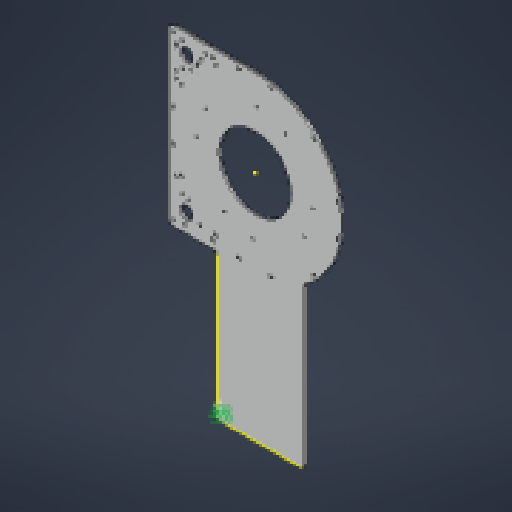
# Autodesk Inventor part: PLATE,SHOOTER,MOUNT
Saved by Autodesk Inventor 2026 (Build 300175000, 175)
## iProperties
Created: 2026-02-09
Part Number: PLATE,SHOOTER,MOUNT
Material: Aluminum 6061
Document SubType Name: Sheet Metal
Designer: littl
Density: 2.7 g/cm^3
Sheet Metal Rule: Default
Appearance: Aluminum - Flat
Mass: 776.002 g
Surface Area: 1574.73 cm^2
Volume: 287.408 cm^3
Author: littl
Autodesk Inventor part; units mm, degrees
ref_plane "YZ Plane" through (0, 0, 0) normal (1, 0, 0) x (0, 1, 0)
ref_plane "XZ Plane" through (0, 0, 0) normal (0, 1, 0) x (-1, 0, 0)
ref_plane "XY Plane" through (0, 0, 0) normal (0, 0, 1) x (1, 0, 0)
sketch "Sketch1" plane through (0, 0, 0) normal (0, 0, 1) x (1, 0, 0)
  line L0 (-190.5, -190.5) -> (190.5, -190.5)
  line L1 (190.5, -190.5) -> (190.5, 190.5)
  line L2 (190.5, 190.5) -> (-190.5, 190.5)
  line L3 (-190.5, 190.5) -> (-190.5, -190.5)
  line L4 (-190.5, -190.5) -> (190.5, 190.5) construction
  line L5 (190.5, -190.5) -> (-190.5, 190.5) construction
  circle A0 centre (0, 0) radius 79.375
  line L6 (130.599, -90.0738) -> (-0.5713, 156.6217) construction
  line L7 (-0.5713, 156.6217) -> (-129.5258, 88.0554) construction
  line L8 (-129.5258, 88.0554) -> (1.6445, -158.6401) construction
  line L9 (1.6445, -158.6401) -> (130.599, -90.0738) construction
  line L10 (130.599, -90.0738) -> (-129.5258, 88.0554) construction
  line L11 (-0.5713, 156.6217) -> (1.6445, -158.6401) construction
  line L12 (1.6445, -158.6401) -> (-64.4772, -34.2832) construction
  line L13 (-64.4772, -34.2832) -> (-12.5828, -6.6904) construction
  line L14 (-65.0486, 122.3386) -> (66.1218, -124.357) construction
  line L15 (-91.2837, -21.0636) -> (-75.8652, -12.8655) construction
  line L16 (-91.2837, -21.0636) -> (-85.3214, -32.2771) construction
  line L17 (-85.3214, -32.2771) -> (-79.3591, -43.4905) construction
  line L18 (68.5077, 63.899) -> (53.0893, 55.7008) construction
  line L19 (68.5077, 63.899) -> (74.47, 52.6855) construction
  line L20 (74.47, 52.6855) -> (80.4323, 41.4721) construction
  arc A1 (0, -190.5) -> (190.5, 0) centre (0, 0) ccw
  arc A2 (190.5, 0) -> (0, 190.5) centre (0, 0) ccw
  point P0 (0.5366, -1.0092)
  point P1 (152.4, 190.5)
  point P2 (-17.6976, -190.5)
  dimension "d0" = 381
  dimension "d1" = 158.75
  dimension "d2" = 279.4
  dimension "d3" = 146.05
  dimension "d4" = 28
  dimension "d5" = 140.843
  dimension "d6" = 114.3
  dimension "d7" = 17.4625
  dimension "d8" = 12.7
  dimension "d9" = 114.3
  dimension "d11" = 17.4625
  dimension "d12" = 12.7
  constraints: 42 end point, 9 midpoint, 7 coincident, 7 point on line, 6 parallel, 5 perpendicular, 4 point on circle, 3 centre point, 3 equal length, 2 collinear, 1 horizontal
  measures "d0" distance of L2.end L1.end
  measures "d1" diameter of A0
  measures "d2" distance of L6.start L6.end
  measures "d3" distance of L6.end L7.end
  measures "d4" angle of L3 L8
  measures "d5" distance of L8.end L12.end
  measures "d6" distance between parallel lines of L7 L15
  measures "d7" distance of L15.start L15.end
  measures "d8" distance of L15.start L16.end
  measures "d9" distance between parallel lines of L7 L18
  measures "d11" distance of L18.start L18.end
  measures "d12" distance of L19.end L20.end
extrude "Plate1" add sketch "Sketch1" along normal blind 4.7752 contours L3 L2 A2 A1 L0
fillet "Corner Round1" radius 12.7 2 edges at (-190.5, 190.5, 2.3876) (-190.5, -190.5, 2.3876)
sketch "Sketch7" plane through (0, 0, 4.7752) normal (0, 0, 1) x (1, 0, 0)
  line L0 (0, 0) -> (-126.9226, 4.4322) construction
  line L1 (0, 266.7) -> (0, -266.7) projected
  circle A0 centre (-79.3591, -43.4905) radius 2.4892 projected
  circle A1 centre (80.4323, 41.4721) radius 2.4892 projected
  line L2 (59.6229, -112.1343) -> (0, 0) construction
  circle A2 centre (-91.2837, -21.0636) radius 2.4892 projected
  circle A3 centre (68.5077, 63.899) radius 2.4892 projected
  line L3 (-91.2837, -21.0636) -> (-79.3591, -43.4905) construction
  line L4 (68.5077, 63.899) -> (80.4323, 41.4721) construction
  point P0 (-112.1343, -59.6229)
  point P1 (-67.2997, -107.7021)
  point P2 (-4.4322, -126.9226)
  point P3 (107.7021, -67.2997)
  point P4 (126.9226, -4.4322)
  point P5 (112.1343, 59.6229)
  point P6 (67.2997, 107.7021)
  point P7 (4.4322, 126.9226)
  point P8 (-59.6229, 112.1343)
  point P9 (-107.7021, 67.2997)
  dimension "d94" = 127
  dimension "d98" = 360
  constraints: 8 end point, 1 parallel, 13 other
  measures "d94" distance of L0.start L0.end
hole "Hole6" at (-126.9226, 4.4322, 4.7752) at (-67.2997, -107.7021, 4.7752) at (-4.4322, -126.9226, 4.7752) at (107.7021, -67.2997, 4.7752) at (126.9226, -4.4322, 4.7752) at (4.4322, 126.9226, 4.7752) at (67.2997, 107.7021, 4.7752) at (-107.7021, 67.2997, 4.7752) direction (0, 0, -1) diameter 4.9784 end through all thread size "1/4-20 UNC" class "2B" standard "ANSI Unified Screw Threads"
sketch "Sketch8" plane through (0, 0, 4.7752) normal (0, 0, 1) x (1, 0, 0)
  circle A0 centre (0, 0) radius 190.5 construction
  arc A1 (-177.8, 190.5) -> (-190.5, 177.8) centre (-177.8, 177.8) ccw projected
  line L0 (-177.8, 177.8) -> (0, 0) construction
  arc A2 (-190.5, -177.8) -> (-177.8, -190.5) centre (-177.8, -177.8) ccw projected
  line L1 (0, 0) -> (-177.8, -177.8) construction
  line L2 (-149.9703, -149.9703) -> (-172.4209, -172.4209) construction
  line L3 (-149.0723, 149.0723) -> (-171.5229, 171.5229) construction
  line L4 (-149.0723, 149.0723) -> (-123.9351, 145.4275) construction
  line L5 (-149.0723, 149.0723) -> (-128.558, 149.0723) construction
  line L6 (-149.9703, -149.9703) -> (-145.5596, -124.9562) construction
  line L7 (-149.9703, -149.9703) -> (-130.8542, -149.9703)
  line L8 (-177.8, 190.5) -> (0, 190.5) projected
  line L9 (-190.5, -177.8) -> (-190.5, 177.8) projected
  line L10 (0, -190.5) -> (-177.8, -190.5) projected
  point P0 (-119.3021, -158.1878)
  point P1 (-158.1878, -119.3021)
  point P2 (-157.2898, 118.4041)
  point P3 (-118.4041, 157.2898)
  point P4 (-174.2094, 152.717)
  point P5 (-154.3809, -174.9844)
  point P6 (-178.698, -178.698)
  dimension "d107" = 381
  dimension "d108" = 212.09
  dimension "d109" = 210.82
  dimension "d110" = 31.75
  dimension "d113" = 360
  dimension "d115" = 31.75
  dimension "d118" = 360
  dimension "d134" = 25.4
  dimension "d137" = 360
  dimension "d139" = 8.25
  dimension "d149" = 360
  dimension "d151" = 25.4
  dimension "d153" = 80
  dimension "d221" = 12.7
  dimension "d222" = 12.7
  dimension "d225" = 40.6272
  constraints: 16 end point, 3 point on line, 2 coincident, 2 collinear, 2 horizontal, 1 centre point, 1 perpendicular, 14 other
  measures "d107" diameter of A0
  measures "d108" distance of point (0, 0) L2.start
  measures "d109" distance of point (0, 0) L3.start
  measures "d110" distance of L2.start L2.end
  measures "d115" distance of L3.start L3.end
  measures "d134" distance of L3.start L4.end
  measures "d139" angle of L4 L5
  measures "d151" distance of L2.start L6.end
  measures "d153" angle of L7 L6
  measures "d221" distance from line of L8 point (-177.8, 177.8)
  measures "d222" distance from line of L9 point (-177.8, 177.8)
  measures "d225" distance of L2.start point (-178.698, -178.698)
hole "Hole7" at (-118.4041, 157.2898, 4.7752) at (-157.2898, 118.4041, 4.7752) at (-177.8, 177.8, 4.7752) at (-158.1878, -119.3021, 4.7752) at (-119.3021, -158.1878, 4.7752) at (-154.3809, -174.9844, 4.7752) at (-174.2094, 152.717, 4.7752) at (-178.698, -178.698, 4.7752) direction (0, 0, -1) diameter 6.5278 depth 4.7752 tip angle 118 clearance for "Flat Head Machine Screw (82)" size "1/4" standard "Ansi Unified Screw Threads"
hole "Hole8" at (-149.0723, 149.0723, 4.7752) at (-149.9703, -149.9703, 4.7752) direction (0, 0, -1) diameter 28.575 depth 4.7752 tip angle 118
hole "Hole9" at (-123.9351, 145.4275, 4.7752) at (-174.2094, 152.717, 4.7752) at (-154.3809, -174.9844, 4.7752) at (-145.5596, -124.9562, 4.7752) direction (0, 0, -1) diameter 4.9784 end through all clearance for "Flat Head Machine Screw (82)" size "#10" standard "Ansi Unified Screw Threads"
sketch "Sketch11" plane through (0, 0, 4.7752) normal (0, 0, 1) x (1, 0, 0)
  line L0 (179.674, -32.5022) -> (178.4352, -38.7302) construction
  line L1 (178.117, -32.1925) -> (176.8782, -38.4205)
  line L2 (179.9922, -39.0399) -> (181.231, -32.8119)
  arc A0 (181.231, -32.8119) -> (178.117, -32.1925) centre (179.674, -32.5022) ccw
  arc A1 (176.8782, -38.4205) -> (179.9922, -39.0399) centre (178.4352, -38.7302) ccw
  line L3 (179.0546, -35.6162) -> (0, 0) construction
  line L4 (-274.701, 0) -> (274.701, 0) construction
  line L5 (162.5024, -83.2593) -> (159.5091, -88.8595) construction
  line L6 (161.1024, -82.5109) -> (158.109, -88.1111)
  line L7 (160.9091, -89.6078) -> (163.9025, -84.0076)
  arc A2 (163.9025, -84.0076) -> (161.1024, -82.5109) centre (162.5024, -83.2593) ccw
  arc A3 (158.109, -88.1111) -> (160.9091, -89.6078) centre (159.5091, -88.8595) ccw
  line L8 (131.3362, -126.8461) -> (126.8461, -131.3362) construction
  line L9 (130.2137, -125.7236) -> (125.7236, -130.2137)
  line L10 (127.9686, -132.4588) -> (132.4588, -127.9686)
  arc A4 (132.4588, -127.9686) -> (130.2137, -125.7236) centre (131.3362, -126.8461) ccw
  arc A5 (125.7236, -130.2137) -> (127.9686, -132.4588) centre (126.8461, -131.3362) ccw
  line L11 (88.8595, -159.5091) -> (83.2593, -162.5024) construction
  line L12 (88.1111, -158.109) -> (82.5109, -161.1024)
  line L13 (84.0076, -163.9025) -> (89.6078, -160.9091)
  arc A6 (89.6078, -160.9091) -> (88.1111, -158.109) centre (88.8595, -159.5091) ccw
  arc A7 (82.5109, -161.1024) -> (84.0076, -163.9025) centre (83.2593, -162.5024) ccw
  line L14 (38.7302, -178.4352) -> (32.5022, -179.674) construction
  line L15 (38.4205, -176.8782) -> (32.1925, -178.117)
  line L16 (32.8119, -181.231) -> (39.0399, -179.9922)
  arc A8 (39.0399, -179.9922) -> (38.4205, -176.8782) centre (38.7302, -178.4352) ccw
  arc A9 (32.1925, -178.117) -> (32.8119, -181.231) centre (32.5022, -179.674) ccw
  arc A10 (84.0076, 163.9025) -> (82.5109, 161.1024) centre (83.2593, 162.5024) ccw
  line L17 (82.5109, 161.1024) -> (88.1111, 158.109)
  line L18 (83.2593, 162.5024) -> (88.8595, 159.5091) construction
  line L19 (89.6078, 160.9091) -> (84.0076, 163.9025)
  arc A11 (88.1111, 158.109) -> (89.6078, 160.9091) centre (88.8595, 159.5091) ccw
  arc A12 (127.9686, 132.4588) -> (125.7236, 130.2137) centre (126.8461, 131.3362) ccw
  line L20 (125.7236, 130.2137) -> (130.2137, 125.7236)
  line L21 (126.8461, 131.3362) -> (131.3362, 126.8461) construction
  line L22 (132.4588, 127.9686) -> (127.9686, 132.4588)
  arc A13 (130.2137, 125.7236) -> (132.4588, 127.9686) centre (131.3362, 126.8461) ccw
  arc A14 (160.9091, 89.6078) -> (158.109, 88.1111) centre (159.5091, 88.8595) ccw
  line L23 (158.109, 88.1111) -> (161.1024, 82.5109)
  line L24 (159.5091, 88.8595) -> (162.5024, 83.2593) construction
  line L25 (163.9025, 84.0076) -> (160.9091, 89.6078)
  arc A15 (179.9922, 39.0399) -> (176.8782, 38.4205) centre (178.4352, 38.7302) ccw
  line L26 (176.8782, 38.4205) -> (178.117, 32.1925)
  line L27 (178.4352, 38.7302) -> (179.674, 32.5022) construction
  line L28 (181.231, 32.8119) -> (179.9922, 39.0399)
  arc A16 (178.117, 32.1925) -> (181.231, 32.8119) centre (179.674, 32.5022) ccw
  arc A17 (161.1024, 82.5109) -> (163.9025, 84.0076) centre (162.5024, 83.2593) ccw
  line L29 (32.5022, 179.674) -> (38.7302, 178.4352) construction
  arc A18 (38.4205, 176.8782) -> (39.0399, 179.9922) centre (38.7302, 178.4352) ccw
  line L30 (32.1925, 178.117) -> (38.4205, 176.8782)
  line L31 (39.0399, 179.9922) -> (32.8119, 181.231)
  arc A19 (32.8119, 181.231) -> (32.1925, 178.117) centre (32.5022, 179.674) ccw
  arc A20 (-163.9025, 84.0076) -> (-161.1024, 82.5109) centre (-162.5024, 83.2593) ccw
  line L32 (-161.1024, 82.5109) -> (-158.109, 88.1111)
  line L33 (-162.5024, 83.2593) -> (-159.5091, 88.8595) construction
  line L34 (-160.9091, 89.6078) -> (-163.9025, 84.0076)
  arc A21 (-158.109, 88.1111) -> (-160.9091, 89.6078) centre (-159.5091, 88.8595) ccw
  arc A22 (-132.4588, 127.9686) -> (-130.2137, 125.7236) centre (-131.3362, 126.8461) ccw
  line L35 (-130.2137, 125.7236) -> (-125.7236, 130.2137)
  line L36 (-131.3362, 126.8461) -> (-126.8461, 131.3362) construction
  line L37 (-127.9686, 132.4588) -> (-132.4588, 127.9686)
  arc A23 (-125.7236, 130.2137) -> (-127.9686, 132.4588) centre (-126.8461, 131.3362) ccw
  arc A24 (-89.6078, 160.9091) -> (-88.1111, 158.109) centre (-88.8595, 159.5091) ccw
  line L38 (-88.1111, 158.109) -> (-82.5109, 161.1024)
  line L39 (-88.8595, 159.5091) -> (-83.2593, 162.5024) construction
  line L40 (-84.0076, 163.9025) -> (-89.6078, 160.9091)
  arc A25 (-39.0399, 179.9922) -> (-38.4205, 176.8782) centre (-38.7302, 178.4352) ccw
  line L41 (-38.4205, 176.8782) -> (-32.1925, 178.117)
  line L42 (-38.7302, 178.4352) -> (-32.5022, 179.674) construction
  line L43 (-32.8119, 181.231) -> (-39.0399, 179.9922)
  arc A26 (-32.1925, 178.117) -> (-32.8119, 181.231) centre (-32.5022, 179.674) ccw
  arc A27 (-82.5109, 161.1024) -> (-84.0076, 163.9025) centre (-83.2593, 162.5024) ccw
  line L44 (-179.674, 32.5022) -> (-178.4352, 38.7302) construction
  arc A28 (-176.8782, 38.4205) -> (-179.9922, 39.0399) centre (-178.4352, 38.7302) ccw
  line L45 (-178.117, 32.1925) -> (-176.8782, 38.4205)
  line L46 (-179.9922, 39.0399) -> (-181.231, 32.8119)
  arc A29 (-181.231, 32.8119) -> (-178.117, 32.1925) centre (-179.674, 32.5022) ccw
  arc A30 (-84.0076, -163.9025) -> (-82.5109, -161.1024) centre (-83.2593, -162.5024) ccw
  line L47 (-82.5109, -161.1024) -> (-88.1111, -158.109)
  line L48 (-83.2593, -162.5024) -> (-88.8595, -159.5091) construction
  line L49 (-89.6078, -160.9091) -> (-84.0076, -163.9025)
  arc A31 (-88.1111, -158.109) -> (-89.6078, -160.9091) centre (-88.8595, -159.5091) ccw
  arc A32 (-127.9686, -132.4588) -> (-125.7236, -130.2137) centre (-126.8461, -131.3362) ccw
  line L50 (-125.7236, -130.2137) -> (-130.2137, -125.7236)
  line L51 (-126.8461, -131.3362) -> (-131.3362, -126.8461) construction
  line L52 (-132.4588, -127.9686) -> (-127.9686, -132.4588)
  arc A33 (-130.2137, -125.7236) -> (-132.4588, -127.9686) centre (-131.3362, -126.8461) ccw
  arc A34 (-160.9091, -89.6078) -> (-158.109, -88.1111) centre (-159.5091, -88.8595) ccw
  line L53 (-158.109, -88.1111) -> (-161.1024, -82.5109)
  line L54 (-159.5091, -88.8595) -> (-162.5024, -83.2593) construction
  line L55 (-163.9025, -84.0076) -> (-160.9091, -89.6078)
  arc A35 (-179.9922, -39.0399) -> (-176.8782, -38.4205) centre (-178.4352, -38.7302) ccw
  line L56 (-176.8782, -38.4205) -> (-178.117, -32.1925)
  line L57 (-178.4352, -38.7302) -> (-179.674, -32.5022) construction
  line L58 (-181.231, -32.8119) -> (-179.9922, -39.0399)
  arc A36 (-178.117, -32.1925) -> (-181.231, -32.8119) centre (-179.674, -32.5022) ccw
  arc A37 (-161.1024, -82.5109) -> (-163.9025, -84.0076) centre (-162.5024, -83.2593) ccw
  line L59 (-32.5022, -179.674) -> (-38.7302, -178.4352) construction
  arc A38 (-38.4205, -176.8782) -> (-39.0399, -179.9922) centre (-38.7302, -178.4352) ccw
  line L60 (-32.1925, -178.117) -> (-38.4205, -176.8782)
  line L61 (-39.0399, -179.9922) -> (-32.8119, -181.231)
  arc A39 (-32.8119, -181.231) -> (-32.1925, -178.117) centre (-32.5022, -179.674) ccw
  line L62 (-95.2952, 171.5495) -> (-89.695, 174.5429) construction
  line L63 (-96.0436, 172.9495) -> (-90.4434, 175.9429)
  line L64 (-88.9467, 173.1428) -> (-94.5469, 170.1494)
  arc A40 (-96.0436, 172.9495) -> (-94.5469, 170.1494) centre (-95.2952, 171.5495) ccw
  arc A41 (-88.9467, 173.1428) -> (-90.4434, 175.9429) centre (-89.695, 174.5429) ccw
  line L65 (-174.5429, 89.695) -> (-171.5495, 95.2952) construction
  line L66 (-175.9429, 90.4434) -> (-172.9495, 96.0436)
  line L67 (-170.1494, 94.5469) -> (-173.1428, 88.9467)
  arc A42 (-175.9429, 90.4434) -> (-173.1428, 88.9467) centre (-174.5429, 89.695) ccw
  arc A43 (-170.1494, 94.5469) -> (-172.9495, 96.0436) centre (-171.5495, 95.2952) ccw
  line L68 (-174.5429, -89.695) -> (-171.5495, -95.2952) construction
  line L69 (-173.1428, -88.9467) -> (-170.1494, -94.5469)
  line L70 (-172.9495, -96.0436) -> (-175.9429, -90.4434)
  arc A44 (-173.1428, -88.9467) -> (-175.9429, -90.4434) centre (-174.5429, -89.695) ccw
  arc A45 (-172.9495, -96.0436) -> (-170.1494, -94.5469) centre (-171.5495, -95.2952) ccw
  line L71 (-95.2952, -171.5495) -> (-89.695, -174.5429) construction
  line L72 (-94.5469, -170.1494) -> (-88.9467, -173.1428)
  line L73 (-90.4434, -175.9429) -> (-96.0436, -172.9495)
  arc A46 (-94.5469, -170.1494) -> (-96.0436, -172.9495) centre (-95.2952, -171.5495) ccw
  arc A47 (-90.4434, -175.9429) -> (-88.9467, -173.1428) centre (-89.695, -174.5429) ccw
  circle A48 centre (0, 0) radius 196.215 construction
  line L74 (0, 0) -> (-92.4951, 173.0462) construction
  line L75 (0, 0) -> (-173.0462, 92.4951) construction
  line L76 (0, 0) -> (-173.0462, -92.4951) construction
  line L77 (0, 0) -> (-92.4951, -173.0462) construction
  point P0 (161.0058, -86.0594)
  point P1 (129.0912, -129.0912)
  point P2 (86.0594, -161.0058)
  point P3 (35.6162, -179.0546)
  point P4 (86.0594, 161.0058)
  point P5 (129.0912, 129.0912)
  point P6 (161.0058, 86.0594)
  point P7 (179.0546, 35.6162)
  point P8 (35.6162, 179.0546)
  point P9 (-161.0058, 86.0594)
  point P10 (-129.0912, 129.0912)
  point P11 (-86.0594, 161.0058)
  point P12 (-35.6162, 179.0546)
  point P13 (-179.0546, 35.6162)
  point P14 (-86.0594, -161.0058)
  point P15 (-129.0912, -129.0912)
  point P16 (-161.0058, -86.0594)
  point P17 (-179.0546, -35.6162)
  point P18 (-35.6162, -179.0546)
  point P19 (-86.0594, 161.0058)
  point P20 (-86.0594, -161.0058)
  dimension "d183" = 3.175
  dimension "d184" = 3.175
  dimension "d185" = 11.25
  dimension "d186" = 182.5625
  dimension "d189" = 67.5
  dimension "d193" = 360
  dimension "d226" = 392.43
  constraints: 202 end point, 100 point on circle, 49 centre point, 20 tangent, 9 parallel, 7 midpoint, 7 perpendicular, 4 equal radius, 2 point on line, 1 coincident, 290 other
  measures "d183" distance of L3.start L0.end
  measures "d184" diameter of A1
  measures "d185" angle of L4 L3
  measures "d186" distance of L3.start L3.end
  measures "d226" diameter of A48
extrude "Cut2" cut sketch "Sketch11" against normal blind 4.7752 contours A0 L2 A1 L1 | A4 L10 A5 L9 | A8 L16 A9 L15 | L22 A13 L20 A12 | L28 A16 L26 A15 | L30 A19 L31 A18 | L34 A21 L32 A20 | L40 A27 L38 A24 | L43 A26 L41 A25 | L45 A29 L46 A28 | L49 A31 L47 A30 | L55 A37 L53 A34 | L58 A36 L56 A35 | L60 A39 L61 A38 | L63 A41 L64 A40 | L66 A43 L67 A42 | L69 A45 L70 A44 | L72 A47 L73 A46
sketch "Sketch13" plane through (0, 0, 4.7752) normal (0, 0, 1) x (1, 0, 0)
  line L0 (0, 0) -> (-107.6796, 172.3234) construction
  line L1 (-172.3234, 107.6796) -> (0, 0) construction
  line L2 (0, 0) -> (-199.0407, 199.0407) construction
  line L3 (0, -268.4081) -> (0, 276.9489) construction
  dimension "d232" = 45
  dimension "d233" = 13
  dimension "d234" = 203.2
  constraints: 6 end point, 1 symmetric about line
  measures "d232" angle of L2 L3
  measures "d233" angle of L2 L0
  measures "d234" distance of L0.start L0.end
hole "Hole13" at (-107.6796, 172.3234, 4.7752) at (-172.3234, 107.6796, 4.7752) direction (0, 0, -1) diameter 6.5278 end through all clearance for "Flat Head Machine Screw (82)" size "1/4" standard "Ansi Unified Screw Threads"
sketch "Sketch14" plane through (0, 0, 0) normal (0, 0, -1) x (-1, 0, 0)
  line L0 (82.55, -190.5) -> (82.55, -508)
  line L1 (190.5, -177.8) -> (190.5, 177.8)
  line L2 (-107.95, -156.9619) -> (-107.95, -508)
  line L3 (82.55, -508) -> (-107.95, -508)
  line L4 (177.8, -190.5) -> (0, -190.5)
  arc A0 (0, 190.5) -> (0, -190.5) centre (0, 0) ccw
  dimension "d242" = 107.95
  dimension "d243" = 190.5
  dimension "d249" = 317.5
  measures "d242" distance between parallel lines of L1 L0
  measures "d243" distance between parallel lines of L0 L2
  measures "d249" distance of L0.start L0.end
sheet face with bend "Face2" sketch "Sketch14" thickness 4.7752 toward (0, 0, 1) bend radius 4.7752 relief straight relief width 4.7752 relief depth 2.3876
bend "Bend1"
sketch "Sketch15" plane through (0, 0, 4.7752) normal (0, 0, 1) x (1, 0, 0)
  circle A0 centre (-149.0723, 149.0723) radius 14.2875 projected
  circle A1 centre (-172.5388, 158.7924) radius 2.4892 projected
  point P0 (0, 0)
  point P1 (-172.5388, 139.3521)
  point P2 (-158.7924, 125.6057)
  point P3 (-139.3521, 125.6057)
  point P4 (-125.6057, 139.3521)
  point P5 (-125.6057, 158.7924)
  point P6 (-139.3521, 172.5388)
  point P7 (-158.7924, 172.5388)
  dimension "d253" = 360
  constraints: 1 coincident, 9 other
hole "Hole14" at (-172.5388, 158.7924, 4.7752) at (-139.3521, 125.6057, 4.7752) at (-125.6057, 139.3521, 4.7752) at (-158.7924, 172.5388, 4.7752) direction (0, 0, -1) diameter 6.35 depth 4.7752 tip angle 118
fillet "Corner Round3" radius 6.35 6 edges at (-172.723, 155.6228, 2.3876) (-174.0011, 155.9742, 2.3876) (-82.55, -190.5, 2.3876) (107.95, -156.9619, 2.3876) (107.95, -508, 2.3876) (-82.55, -508, 2.3876)
sketch "Sketch16" plane through (0, 0, 4.7752) normal (0, 0, 1) x (1, 0, 0)
  point P0 (0, 0)
sketch "Sketch17" plane through (0, 0, 4.7752) normal (0, 0, 1) x (1, 0, 0)
  line L0 (101.6, -508) -> (-76.2, -508) projected
  line L1 (-82.55, -501.65) -> (-82.55, -196.85) projected
  point P0 (0, 0)
  point P1 (-73.025, -495.3)
  point P2 (-73.025, -482.6)
  dimension "d263" = 12.7
  dimension "d264" = 12.7
  dimension "d265" = 9.525
  constraints: 1 vertical alignment
  measures "d263" distance of point (-73.025, -495.3) point (-73.025, -482.6)
  measures "d264" distance from line of L0 point (-73.025, -495.3)
  measures "d265" distance from line of L1 point (-73.025, -495.3)
equation "\"d11\" = d7"
equation "\"d105\" = Thickness"
equation "\"d125\" = Thickness"
equation "\"d132\" = Thickness"
equation "\"d13\" = Thickness"
equation "\"BendRadius\" = Thickness"
equation "\"BendReliefWidth\" = Thickness"
equation "\"BendReliefDepth\" = 0.5 * Thickness"
equation "\"CornerReliefSize\" = 4 * Thickness"
equation "\"MinimumRemnant\" = 2 * Thickness"
equation "\"TransitionRadius\" = BendRadius"
equation "\"JacobiRadiusSize\" = BendRadius"
equation "\"GapSize\" = Thickness"
equation "\"Thickness\" = 4.7752"
body "Solid1"
